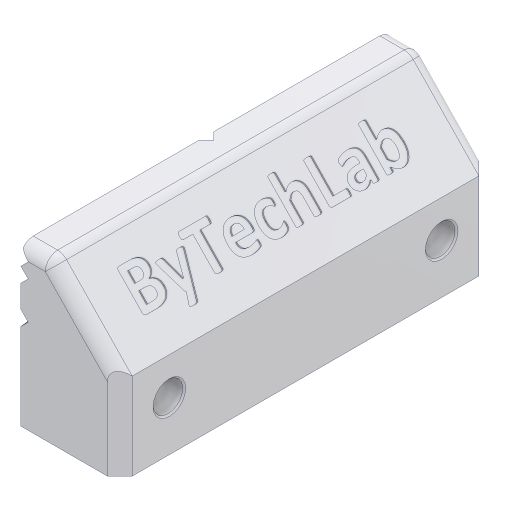
# Autodesk Inventor part: 3DP_ABS_Jaw_First_Half
Saved by Autodesk Inventor 2024.3 (Build 283343000, 343)
## iProperties
Created: 2018-02-17
Part Number: 3DP_ABS_Jaw_First_Half
Material: Ogólny
Document SubType Name: Modeling
Designer: Andrzej
Density: 1 g/cm^3
Appearance: PTFE
Author: Andrzej
Autodesk Inventor part; units mm, degrees
ref_plane "YZ Plane" through (0, 0, 0) normal (1, 0, 0) x (0, 1, 0)
ref_plane "XZ Plane" through (0, 0, 0) normal (0, 1, 0) x (-1, 0, 0)
ref_plane "XY Plane" through (0, 0, 0) normal (0, 0, 1) x (1, 0, 0)
sketch "Szkic1" plane through (0, 0, 0) normal (0, 0, 1) x (1, 0, 0)
  line L0 (-10, 37.5) -> (10, 37.5)
  line L1 (10, 37.5) -> (10, -37.5)
  line L2 (10, -37.5) -> (-10, -37.5)
  line L3 (-10, -37.5) -> (-10, 37.5)
  point P0 (0, 0)
  dimension "d0" = 20
  dimension "d1" = 75
  dimension "d39" = 37.5
  dimension "d40" = 10
  constraints: 8 end point, 2 parallel, 1 horizontal, 1 perpendicular
  measures "d0" distance of L1.end L2.end
  measures "d1" distance of L0.end L1.end
  measures "d39" distance from line of point (0, 0) L0
  measures "d40" distance from line of point (0, 0) L1
extrude "Wyciągnięcie proste1" add sketch "Szkic1" along normal blind 32
sketch "Szkic2" plane through (10, -37.5, 0) normal (1, 0, 0) x (0, 0, -1)
  line L0 (0, 75) -> (0, 0) projected
  line L1 (0, 75) -> (-32, 75) projected
  line L2 (-32, 0) -> (-32, 75) projected
  line L3 (0, 0) -> (-32, 0) projected
  point P0 (0, 37.5)
  point P1 (-10, 10)
  point P2 (-10, 65)
  dimension "d4" = 32
  dimension "d5" = 10
  dimension "d6" = 10
  dimension "d7" = 10
  dimension "d8" = 10
  measures "d4" distance of L0.end L2.start
  measures "d5" distance from line of L0 point (-10, 10)
  measures "d6" distance from line of L0 point (-10, 65)
  measures "d7" distance from line of L3 point (-10, 10)
  measures "d8" distance from line of L1 point (-10, 65)
hole "Otwór1" at (10, -27.5, 10) at (10, 27.5, 10) direction (-1, 0, 0) diameter 6 end through all
sketch "Szkic3" plane through (-10, 37.5, 0) normal (0, 1, 0) x (1, 0, 0)
  line L0 (0, 0) -> (20, 0) projected
  line L1 (0, 0) -> (0, -32) projected
  line L2 (20, -32) -> (0, -32) projected
  line L3 (20, 0) -> (20, -32) projected
  line L4 (0, -28) -> (1.5, -26.5)
  line L5 (0, -28) -> (2.2095, -28) construction
  line L6 (0, 0) -> (0, -32) projected
  line L7 (0, -25) -> (1.5, -26.5)
  line L8 (0, -25) -> (2.7592, -25) construction
  dimension "d17" = 45
  dimension "d19" = 45
  dimension "d20" = 3
  dimension "d21" = 4
  constraints: 8 end point, 2 horizontal, 2 point on line
  measures "d17" angle of L5 L4
  measures "d19" angle of L7 L8
  measures "d20" distance of L7.start L4.start
  measures "d21" distance from line of L2 L4.start
extrude "Wyciągnięcie proste2" cut sketch "Szkic3" against normal through all contours L7 L4 L1
chamfer "Faza1" distance 14 distance2 14.5 1 edges at (10, 0, 32) measured on face at (9.5, 0, 32)
chamfer "Faza2" distance 2.5 angle 45 2 edges at (10, -37.5, 8.75) (10, 37.5, 8.75)
ref_plane "Płaszczyzna konstrukcyjna1" through (-10, 37.5, 32) normal (0, -0.9902681, -0.1391731) x (-1, 0, 0)
sketch "Szkic4" plane through (-10, 37.5, 32) normal (0, -0.9902681, -0.1391731) x (-1, 0, 0)
  line L0 (-17.5, 31.6886) -> (-17.5, 11.7948) projected
  line L1 (0, 31.6886) -> (-17.5, 31.6886) projected
  line L2 (0, 31.6886) -> (0, 6.9319) projected
  line L3 (0, 6.9319) -> (-1.5, 5.4465) projected
  line L4 (-1.5, 5.4465) -> (0, 3.9611) projected
  line L5 (0, 3.9611) -> (0, 0) projected
  line L6 (-6, 0) -> (0, 0) projected
  line L7 (-17.5, 11.7948) -> (-6, 0) projected
  line L8 (0, -3.5061) -> (0, 6.9319) projected
  line L9 (0, 1) -> (-1.5, 2.5)
  line L10 (0, 1) -> (2.5951, 1) construction
  line L11 (0, 31.6886) -> (0, 6.9319) projected
  line L12 (0, 4) -> (-1.5, 2.5)
  line L13 (0, 4) -> (3.5979, 4) construction
  line L14 (0, 1) -> (0, 4)
  point P0 (-10, 26.4696)
  dimension "d32" = 135
  dimension "d34" = 135
  dimension "d35" = 3
  dimension "d36" = 1
  constraints: 10 end point, 2 horizontal, 2 point on line, 1 collinear
  measures "d32" angle of L10 L9
  measures "d34" angle of L12 L13
  measures "d35" distance of L12.start L9.start
  measures "d36" distance of L5.end L9.start
extrude "Wyciągnięcie proste3" cut sketch "Szkic4" along normal through all contours L8 L4 L12 | L9 L12 L4 L5
mirror "Odbicie lustrzane1" about plane through (0, 0, 0) normal (0, 1, 0) of "Wyciągnięcie proste3"
sketch "Szkic5" plane through (0, 0, 32) normal (0, 0, 1) x (1, 0, 0)
  line L0 (-4, 37.5) -> (-4, -37.5) projected
  line L1 (-4, 37.5) -> (-10, 37.5) projected
  line L2 (-10, 37.5) -> (-10, -37.5) projected
  line L3 (-10, -37.5) -> (-4, -37.5) projected
  line L4 (-10, 1.5) -> (-4.369, 1.5) construction
  line L5 (-10, -37.5) -> (-10, 0) projected
  line L6 (-10, -1.5) -> (-2.768, -1.5) construction
  line L7 (-10, -1.5) -> (-8.5, 0)
  line L8 (-10, 1.5) -> (-8.5, 0)
  point P0 (0, 0)
  dimension "d45" = 3
  dimension "d46" = 45
  dimension "d47" = 45
  dimension "d48" = 75
  dimension "d49" = 36
  constraints: 8 end point, 2 horizontal, 2 point on line, 1 perpendicular
  measures "d45" distance of L6.start L4.start
  measures "d46" angle of L4 L8
  measures "d47" angle of L6 L7
  measures "d48" distance of L1.end L2.end
  measures "d49" distance from line of L1 L4.start
extrude "Wyciągnięcie proste4" cut sketch "Szkic5" against normal through all contours L8 L7 L2
fillet "Zaokrąglenie1" radius 2.5 5 edges at (-4, 0, 32) (1.75, 37.5, 26.0446) (1.75, -37.5, 26.0446) (-7, -37.5, 32) (-7, 37.5, 32)
sketch "Szkic6" plane through (-10, 37.5, 0) normal (-1, 0, 0) x (0, 0, 1)
  line L0 (0, -36) -> (22.4796, -36) projected
  line L1 (22.4796, -36) -> (17.4201, 0) projected
  line L2 (0, 0) -> (17.4201, 0) projected
  line L3 (0, -36) -> (0, 0) projected
  circle A0 centre (10, -10) radius 3 projected
  line L4 (22.4796, -39) -> (0, -39) projected
  line L5 (0, -75) -> (0, -39) projected
  line L6 (0, -75) -> (17.4201, -75) projected
  line L7 (17.4201, -75) -> (22.4796, -39) projected
  circle A1 centre (10, -65) radius 3 projected
  circle A2 centre (10, -10) radius 5
  circle A3 centre (10, -65) radius 5
  line L8 (15, -12.8868) -> (10, -15.7735)
  line L9 (10, -15.7735) -> (5, -12.8868)
  line L10 (5, -12.8868) -> (5, -7.1132)
  line L11 (5, -7.1132) -> (10, -4.2265)
  line L12 (10, -4.2265) -> (15, -7.1132)
  line L13 (15, -7.1132) -> (15, -12.8868)
  line L14 (15, -67.8868) -> (10, -70.7735)
  line L15 (10, -70.7735) -> (5, -67.8868)
  line L16 (5, -67.8868) -> (5, -62.1132)
  line L17 (5, -62.1132) -> (10, -59.2265)
  line L18 (10, -59.2265) -> (15, -62.1132)
  line L19 (15, -62.1132) -> (15, -67.8868)
  point P0 (0, -37.5)
  point P1 (15, -10)
  point P2 (15, -65)
  dimension "d56" = 10
  dimension "d57" = 10
  constraints: 24 end point, 4 coincident, 2 horizontal alignment, 2 midpoint, 1 point on line, 30 other
extrude "Wyciągnięcie proste5" cut sketch "Szkic6" against normal blind 5 contours A2 | L13 L8 A2 | A2 L12 L13 | A2 L11 L12 | L8 L9 A2 | A2 L10 L11 | L9 L10 A2 | A3 | L19 L14 A3 | A3 L18 L19 | A3 L17 L18 | L14 L15 A3 | A3 L16 L17 | L15 L16 A3
chamfer "Faza4" distance 0.3 angle 45 4 edges at (-5, 27.5, 13) (10, 27.5, 13) (-5, -27.5, 13) (10, -27.5, 13)
sketch "Szkic7" plane through (-3.2628, -35, 31.2365) normal (0.7194015, 0, 0.6945945) x (0.6945945, 0, -0.7194015)
  line L0 (0, 70) -> (19.0943, 70) projected
  line L1 (0, 0) -> (0, 70) projected
  line L2 (19.0943, 0) -> (0, 0) projected
  line L3 (19.0943, 0) -> (19.0943, 70) projected
  line L4 (3.9416, 6.0812) -> (3.9416, 71.7325) construction
  line L5 (3.9416, 71.7325) -> (20.2301, 71.7325) construction
  line L6 (20.2301, 71.7325) -> (20.2301, 6.0812) construction
  line L7 (20.2301, 6.0812) -> (3.9416, 6.0812) construction
  spline S0 degree 2 poles (10.1237, 12.7216) (10.5519, 12.7216) (11.243, 12.4887) (11.7688, 12.0756) (12.1519, 11.5047) (12.3923, 10.8136) (12.5125, 10.0324) (12.5125, 9.5516) knots 0 0 0 1 2 3 4 5 6 6 6
  line L8 (12.5125, 9.5516) -> (12.5125, 7.4333)
  spline S1 degree 2 poles (12.5125, 7.4333) (12.5125, 7.2305) (12.2721, 6.9526) (12.0017, 6.9526) knots 0 0 0 1 2 2 2
  line L9 (12.0017, 6.9526) -> (5.0608, 6.9526)
  spline S2 degree 2 poles (5.0608, 6.9526) (4.7904, 6.9526) (4.55, 7.2305) (4.55, 7.4333) knots 0 0 0 1 2 2 2
  line L10 (4.55, 7.4333) -> (4.55, 9.4315)
  spline S3 degree 2 poles (4.55, 9.4315) (4.55, 10.1676) (4.7979, 11.1817) (5.2937, 11.8803) (6.0599, 12.2484) (6.5782, 12.2484) knots 0 0 0 1 2 3 4 4 4
  spline S4 degree 2 poles (6.5782, 12.2484) (6.8636, 12.2484) (7.3744, 12.0981) (7.7951, 11.8202) (8.1181, 11.407) (8.2158, 11.1366) knots 0 0 0 1 2 3 4 4 4
  spline S5 degree 2 poles (8.2158, 11.1366) (8.2759, 11.4822) (8.5838, 12.053) (9.0646, 12.4737) (9.7181, 12.7216) (10.1237, 12.7216) knots 0 0 0 1 2 3 4 4 4
  spline S6 degree 2 poles (10.1763, 11.039) (9.9059, 11.039) (9.4702, 10.8512) (9.1697, 10.4981) (9.012, 9.9422) (9.012, 9.4991) knots 0 0 0 1 2 3 4 4 4
  line L11 (9.012, 9.4991) -> (9.012, 8.5376)
  line L12 (9.012, 8.5376) -> (11.273, 8.5376)
  line L13 (11.273, 8.5376) -> (11.273, 9.7094)
  spline S7 degree 2 poles (11.273, 9.7094) (11.273, 10.0474) (11.1303, 10.5056) (10.8524, 10.8512) (10.4467, 11.039) (10.1763, 11.039) knots 0 0 0 1 2 3 4 4 4
  spline S8 degree 2 poles (6.7735, 10.6333) (6.5331, 10.6333) (6.15, 10.4831) (5.8946, 10.1901) (5.7594, 9.7394) (5.7594, 9.3563) knots 0 0 0 1 2 3 4 4 4
  line L14 (5.7594, 9.3563) -> (5.7594, 8.5376)
  line L15 (5.7594, 8.5376) -> (7.8327, 8.5376)
  line L16 (7.8327, 8.5376) -> (7.8327, 9.4465)
  spline S9 degree 2 poles (7.8327, 9.4465) (7.8327, 9.7995) (7.6674, 10.2202) (7.3744, 10.4981) (6.9838, 10.6333) (6.7735, 10.6333) knots 0 0 0 1 2 3 4 4 4
  line L17 (12.5125, 17.1009) -> (14.458, 16.4399)
  spline S10 degree 2 poles (14.458, 16.4399) (14.6082, 16.3873) (14.7435, 15.8915) (14.7435, 15.4183) knots 0 0 0 1 2 2 2
  spline S11 degree 2 poles (14.7435, 15.4183) (14.7435, 15.1704) (14.6984, 14.8775) (14.6007, 14.7272) (14.458, 14.7122) (14.3528, 14.7573) knots 0 0 0 1 2 3 4 4 4
  line L18 (14.3528, 14.7573) -> (12.5125, 15.4934)
  spline S12 degree 2 poles (12.5125, 15.4934) (12.4749, 15.4108) (12.3247, 15.2831) (12.2345, 15.253) knots 0 0 0 1 2 2 2
  line L19 (12.2345, 15.253) -> (7.1942, 13.3676)
  spline S13 degree 2 poles (7.1942, 13.3676) (6.9763, 13.285) (6.751, 13.285) (6.6233, 13.4352) (6.5707, 13.7807) (6.5707, 14.0737) knots 0 0 0 1 2 3 4 4 4
  spline S14 degree 2 poles (6.5707, 14.0737) (6.5707, 14.3366) (6.5857, 14.6446) (6.6608, 14.8174) (6.8186, 14.9075) (6.9613, 14.9526) knots 0 0 0 1 2 3 4 4 4
  line L20 (6.9613, 14.9526) -> (10.627, 16.2371)
  line L21 (10.627, 16.2371) -> (10.627, 16.2596)
  line L22 (10.627, 16.2596) -> (6.8862, 17.439)
  spline S15 degree 2 poles (6.8862, 17.439) (6.7209, 17.469) (6.6233, 17.5892) (6.5707, 17.8596) (6.5707, 18.1976) knots 0 0 0 1 2 3 3 3
  spline S16 degree 2 poles (6.5707, 18.1976) (6.5707, 18.4606) (6.6233, 18.8136) (6.7585, 18.9789) (6.9838, 18.9789) (7.1341, 18.9338) knots 0 0 0 1 2 3 4 4 4
  line L23 (7.1341, 18.9338) -> (12.5125, 17.1009)
  spline S17 degree 2 poles (5.2111, 25.2812) (5.3913, 25.2812) (5.6467, 25.2512) (5.797, 25.1911) (5.8721, 25.0934) (5.8721, 25.0408) knots 0 0 0 1 2 3 4 4 4
  line L24 (5.8721, 25.0408) -> (5.8721, 23.0502)
  line L25 (5.8721, 23.0502) -> (12.2946, 23.0502)
  spline S18 degree 2 poles (12.2946, 23.0502) (12.3547, 23.0502) (12.4524, 22.9676) (12.5125, 22.7873) (12.55, 22.4718) (12.55, 22.239) knots 0 0 0 1 2 3 4 4 4
  spline S19 degree 2 poles (12.55, 22.239) (12.55, 22.0061) (12.5125, 21.6906) (12.4524, 21.5103) (12.3547, 21.4277) (12.2946, 21.4277) knots 0 0 0 1 2 3 4 4 4
  line L26 (12.2946, 21.4277) -> (5.8721, 21.4277)
  line L27 (5.8721, 21.4277) -> (5.8721, 19.4371)
  spline S20 degree 2 poles (5.8721, 19.4371) (5.8721, 19.377) (5.797, 19.2868) (5.6467, 19.2268) (5.3913, 19.1967) (5.2111, 19.1967) knots 0 0 0 1 2 3 4 4 4
  spline S21 degree 2 poles (5.2111, 19.1967) (5.0308, 19.1967) (4.7679, 19.2268) (4.6176, 19.2868) (4.55, 19.377) (4.55, 19.4371) knots 0 0 0 1 2 3 4 4 4
  line L28 (4.55, 19.4371) -> (4.55, 25.0408)
  spline S22 degree 2 poles (4.55, 25.0408) (4.55, 25.0934) (4.6176, 25.1911) (4.7679, 25.2512) (5.0308, 25.2812) (5.2111, 25.2812) knots 0 0 0 1 2 3 4 4 4
  spline S23 degree 2 poles (9.3951, 31.2155) (9.6805, 31.2155) (9.951, 30.9601) (9.951, 30.7422) knots 0 0 0 1 2 2 2
  line L29 (9.951, 30.7422) -> (9.951, 27.3995)
  spline S24 degree 2 poles (9.951, 27.3995) (10.304, 27.3995) (10.8749, 27.5648) (11.273, 27.9329) (11.4834, 28.5038) (11.4834, 28.9019) knots 0 0 0 1 2 3 4 4 4
  spline S25 degree 2 poles (11.4834, 28.9019) (11.4834, 29.3075) (11.3632, 29.9235) (11.228, 30.3742) (11.1078, 30.6671) (11.1078, 30.7648) knots 0 0 0 1 2 3 4 4 4
  spline S26 degree 2 poles (11.1078, 30.7648) (11.1078, 30.8174) (11.1528, 30.8925) (11.258, 30.9451) (11.4608, 30.9601) (11.6186, 30.9601) knots 0 0 0 1 2 3 4 4 4
  spline S27 degree 2 poles (11.6186, 30.9601) (11.7538, 30.9601) (11.9416, 30.9451) (12.0768, 30.9225) (12.1744, 30.8775) (12.2571, 30.7948) (12.4073, 30.4343) (12.55, 29.8784) (12.6552, 29.1648) (12.6552, 28.7592) knots 0 0 0 1 2 3 4 5 6 7 8 8 8
  spline S28 degree 2 poles (12.6552, 28.7592) (12.6552, 28.0305) (12.2871, 26.9263) (11.5359, 26.1826) (10.3942, 25.8221) (9.6205, 25.8221) knots 0 0 0 1 2 3 4 4 4
  spline S29 degree 2 poles (9.6205, 25.8221) (8.8918, 25.8221) (7.7125, 26.2052) (6.8937, 26.9338) (6.4655, 27.9704) (6.4655, 28.6239) knots 0 0 0 1 2 3 4 4 4
  spline S30 degree 2 poles (6.4655, 28.6239) (6.4655, 29.315) (6.8712, 30.2915) (7.5923, 30.9225) (8.5763, 31.2155) (9.1547, 31.2155) knots 0 0 0 1 2 3 4 4 4
  line L30 (9.1547, 31.2155) -> (9.3951, 31.2155)
  spline S31 degree 2 poles (8.9519, 29.7131) (8.3059, 29.7282) (7.5622, 29.1723) (7.5622, 28.5864) knots 0 0 0 1 2 2 2
  spline S32 degree 2 poles (7.5622, 28.5864) (7.5622, 28.2934) (7.7801, 27.8577) (8.1557, 27.5648) (8.6665, 27.4145) (8.9519, 27.3995) knots 0 0 0 1 2 3 4 4 4
  line L31 (8.9519, 27.3995) -> (8.9519, 29.7131)
  spline S33 degree 2 poles (11.4308, 36.639) (11.5885, 36.639) (11.8064, 36.6239) (11.9566, 36.5864) (12.0467, 36.5488) (12.1895, 36.3986) (12.3923, 36.0455) (12.55, 35.5873) (12.6477, 35.054) (12.6477, 34.7685) knots 0 0 0 1 2 3 4 5 6 7 8 8 8
  spline S34 degree 2 poles (12.6477, 34.7685) (12.6477, 34.1376) (12.2571, 33.1535) (11.4834, 32.4925) (10.3791, 32.1545) (9.658, 32.1545) knots 0 0 0 1 2 3 4 4 4
  spline S35 degree 2 poles (9.658, 32.1545) (8.8392, 32.1545) (7.6374, 32.5676) (6.8486, 33.3038) (6.4655, 34.3103) (6.4655, 34.9188) knots 0 0 0 1 2 3 4 4 4
  spline S36 degree 2 poles (6.4655, 34.9188) (6.4655, 35.1592) (6.5557, 35.6399) (6.6984, 36.0455) (6.8862, 36.3761) (7.0214, 36.5113) (7.1115, 36.5638) (7.2618, 36.5939) (7.4796, 36.6164) (7.6298, 36.6164) knots 0 0 0 1 2 3 4 5 6 7 8 8 8
  spline S37 degree 2 poles (7.6298, 36.6164) (7.9904, 36.6164) (8.2759, 36.4887) (8.2759, 36.3911) knots 0 0 0 1 2 2 2
  spline S38 degree 2 poles (8.2759, 36.3911) (8.2759, 36.2859) (8.1031, 36.053) (7.8928, 35.7376) (7.72, 35.2944) (7.72, 34.9864) knots 0 0 0 1 2 3 4 4 4
  spline S39 degree 2 poles (7.72, 34.9864) (7.72, 34.3779) (8.6514, 33.7394) (9.5528, 33.7394) knots 0 0 0 1 2 2 2
  spline S40 degree 2 poles (9.5528, 33.7394) (9.996, 33.7394) (10.6721, 33.8972) (11.1303, 34.2127) (11.3557, 34.6859) (11.3557, 35.0014) knots 0 0 0 1 2 3 4 4 4
  spline S41 degree 2 poles (11.3557, 35.0014) (11.3557, 35.3244) (11.1679, 35.7826) (10.9275, 36.1282) (10.7397, 36.361) (10.7397, 36.4437) knots 0 0 0 1 2 3 4 4 4
  spline S42 degree 2 poles (10.7397, 36.4437) (10.7397, 36.4962) (10.7998, 36.5714) (10.9651, 36.6164) (11.228, 36.639) (11.4308, 36.639) knots 0 0 0 1 2 3 4 4 4
  spline S43 degree 2 poles (12.3021, 43.0014) (12.3622, 43.0014) (12.4599, 42.9263) (12.52, 42.7535) (12.55, 42.453) (12.55, 42.2277) knots 0 0 0 1 2 3 4 4 4
  spline S44 degree 2 poles (12.55, 42.2277) (12.55, 42.0023) (12.52, 41.7019) (12.4599, 41.5291) (12.3622, 41.454) (12.3021, 41.454) knots 0 0 0 1 2 3 4 4 4
  line L32 (12.3021, 41.454) -> (9.1697, 41.454)
  spline S45 degree 2 poles (9.1697, 41.454) (8.7716, 41.454) (8.3134, 41.3338) (7.9904, 41.116) (7.8101, 40.7629) (7.8101, 40.53) knots 0 0 0 1 2 3 4 4 4
  spline S46 degree 2 poles (7.8101, 40.53) (7.8101, 40.2371) (8.2383, 39.6286) (8.6514, 39.3056) knots 0 0 0 1 2 2 2
  line L33 (8.6514, 39.3056) -> (12.3021, 39.3056)
  spline S47 degree 2 poles (12.3021, 39.3056) (12.3622, 39.3056) (12.4599, 39.2305) (12.52, 39.0502) (12.55, 38.7573) (12.55, 38.5319) knots 0 0 0 1 2 3 4 4 4
  spline S48 degree 2 poles (12.55, 38.5319) (12.55, 38.3066) (12.52, 38.0136) (12.4599, 37.8333) (12.3622, 37.7582) (12.3021, 37.7582) knots 0 0 0 1 2 3 4 4 4
  line L34 (12.3021, 37.7582) -> (4.2045, 37.7582)
  spline S49 degree 2 poles (4.2045, 37.7582) (4.1444, 37.7582) (4.0467, 37.8333) (3.9791, 38.0136) (3.9416, 38.3066) (3.9416, 38.5319) knots 0 0 0 1 2 3 4 4 4
  spline S50 degree 2 poles (3.9416, 38.5319) (3.9416, 38.7573) (3.9791, 39.0502) (4.0467, 39.2305) (4.1444, 39.3056) (4.2045, 39.3056) knots 0 0 0 1 2 3 4 4 4
  line L35 (4.2045, 39.3056) -> (7.2467, 39.3056)
  spline S51 degree 2 poles (7.2467, 39.3056) (6.8561, 39.7038) (6.4655, 40.5376) (6.4655, 40.9883) knots 0 0 0 1 2 2 2
  spline S52 degree 2 poles (6.4655, 40.9883) (6.4655, 41.5441) (6.8336, 42.3178) (7.4721, 42.7911) (8.3284, 43.0014) (8.9369, 43.0014) knots 0 0 0 1 2 3 4 4 4
  line L36 (8.9369, 43.0014) -> (12.3021, 43.0014)
  spline S53 degree 2 poles (11.8364, 48.9958) (12.0167, 48.9958) (12.2721, 48.9657) (12.4374, 48.9056) (12.5125, 48.808) (12.5125, 48.7479) knots 0 0 0 1 2 3 4 4 4
  line L37 (12.5125, 48.7479) -> (12.5125, 45.0972)
  spline S54 degree 2 poles (12.5125, 45.0972) (12.5125, 44.8944) (12.2721, 44.6164) (12.0017, 44.6164) knots 0 0 0 1 2 2 2
  line L38 (12.0017, 44.6164) -> (4.7679, 44.6164)
  spline S55 degree 2 poles (4.7679, 44.6164) (4.7078, 44.6164) (4.6101, 44.6991) (4.55, 44.8793) (4.5125, 45.1948) (4.5125, 45.4277) knots 0 0 0 1 2 3 4 4 4
  spline S56 degree 2 poles (4.5125, 45.4277) (4.5125, 45.6681) (4.55, 45.9761) (4.6101, 46.1563) (4.7078, 46.239) (4.7679, 46.239) knots 0 0 0 1 2 3 4 4 4
  line L39 (4.7679, 46.239) -> (11.1754, 46.239)
  line L40 (11.1754, 46.239) -> (11.1754, 48.7479)
  spline S57 degree 2 poles (11.1754, 48.7479) (11.1754, 48.808) (11.243, 48.9056) (11.4007, 48.9657) (11.6486, 48.9958) (11.8364, 48.9958) knots 0 0 0 1 2 3 4 4 4
  spline S58 degree 2 poles (12.3247, 54.5319) (12.4073, 54.5319) (12.505, 54.4117) (12.55, 54.1413) (12.55, 53.8859) knots 0 0 0 1 2 3 3 3
  spline S59 degree 2 poles (12.55, 53.8859) (12.55, 53.608) (12.505, 53.3601) (12.4073, 53.2549) (12.3247, 53.2549) knots 0 0 0 1 2 3 3 3
  line L41 (12.3247, 53.2549) -> (11.8815, 53.2549)
  spline S60 degree 2 poles (11.8815, 53.2549) (12.2496, 52.9169) (12.6552, 52.0455) (12.6552, 51.5197) knots 0 0 0 1 2 2 2
  spline S61 degree 2 poles (12.6552, 51.5197) (12.6552, 51.0765) (12.4298, 50.3479) (11.9791, 49.807) (11.3181, 49.5141) (10.8749, 49.5141) knots 0 0 0 1 2 3 4 4 4
  spline S62 degree 2 poles (10.8749, 49.5141) (10.3942, 49.5141) (9.6881, 49.8897) (9.2223, 50.6333) (9.0045, 51.7451) (9.0045, 52.4812) knots 0 0 0 1 2 3 4 4 4
  line L42 (9.0045, 52.4812) -> (9.0045, 53.0145)
  line L43 (9.0045, 53.0145) -> (8.674, 53.0145)
  spline S63 degree 2 poles (8.674, 53.0145) (8.4111, 53.0145) (8.0205, 52.9094) (7.7575, 52.669) (7.6374, 52.2709) (7.6374, 51.9704) knots 0 0 0 1 2 3 4 4 4
  spline S64 degree 2 poles (7.6374, 51.9704) (7.6374, 51.5873) (7.8101, 50.9714) (8.0205, 50.5056) (8.1932, 50.1901) (8.1932, 50.0925) knots 0 0 0 1 2 3 4 4 4
  spline S65 degree 2 poles (8.1932, 50.0925) (8.1932, 50.0249) (8.1106, 49.9197) (7.9453, 49.8521) (7.7125, 49.8145) (7.5697, 49.8145) knots 0 0 0 1 2 3 4 4 4
  spline S66 degree 2 poles (7.5697, 49.8145) (7.382, 49.8145) (7.1641, 49.8746) (6.9838, 50.0474) (6.766, 50.4831) (6.5857, 51.0615) (6.4655, 51.7451) (6.4655, 52.1056) knots 0 0 0 1 2 3 4 5 6 6 6
  spline S67 degree 2 poles (6.4655, 52.1056) (6.4655, 52.7516) (6.7209, 53.6681) (7.2392, 54.2615) (8.0655, 54.5319) (8.6289, 54.5319) knots 0 0 0 1 2 3 4 4 4
  line L44 (8.6289, 54.5319) -> (12.3247, 54.5319)
  line L45 (9.9735, 53.0145) -> (9.9735, 52.4211)
  spline S68 degree 2 poles (9.9735, 52.4211) (9.9735, 52.0455) (10.0862, 51.5197) (10.304, 51.1892) (10.6195, 51.0315) (10.8223, 51.0315) knots 0 0 0 1 2 3 4 4 4
  spline S69 degree 2 poles (10.8223, 51.0315) (11.1679, 51.0315) (11.5585, 51.4671) (11.5585, 51.8577) knots 0 0 0 1 2 2 2
  spline S70 degree 2 poles (11.5585, 51.8577) (11.5585, 52.1807) (11.228, 52.7291) (10.905, 53.0145) knots 0 0 0 1 2 2 2
  line L46 (10.905, 53.0145) -> (9.9735, 53.0145)
  spline S71 degree 2 poles (9.4852, 61.6005) (10.2214, 61.6005) (11.3857, 61.2775) (12.212, 60.6765) (12.6552, 59.7976) (12.6552, 59.2343) knots 0 0 0 1 2 3 4 4 4
  spline S72 degree 2 poles (12.6552, 59.2343) (12.6552, 58.9563) (12.55, 58.4756) (12.3172, 58.0399) (11.9566, 57.6117) (11.7087, 57.3939) knots 0 0 0 1 2 3 4 4 4
  line L47 (11.7087, 57.3939) -> (12.3021, 57.3939)
  spline S73 degree 2 poles (12.3021, 57.3939) (12.3697, 57.3939) (12.4674, 57.3263) (12.5275, 57.1685) (12.55, 56.9131) (12.55, 56.7253) knots 0 0 0 1 2 3 4 4 4
  spline S74 degree 2 poles (12.55, 56.7253) (12.55, 56.5376) (12.5275, 56.2897) (12.4674, 56.1319) (12.3697, 56.0718) (12.3021, 56.0718) knots 0 0 0 1 2 3 4 4 4
  line L48 (12.3021, 56.0718) -> (4.2045, 56.0718)
  spline S75 degree 2 poles (4.2045, 56.0718) (4.1444, 56.0718) (4.0467, 56.1469) (3.9791, 56.3272) (3.9416, 56.6202) (3.9416, 56.8455) knots 0 0 0 1 2 3 4 4 4
  spline S76 degree 2 poles (3.9416, 56.8455) (3.9416, 57.0709) (3.9791, 57.3638) (4.0467, 57.5441) (4.1444, 57.6192) (4.2045, 57.6192) knots 0 0 0 1 2 3 4 4 4
  line L49 (4.2045, 57.6192) -> (7.2467, 57.6192)
  spline S77 degree 2 poles (7.2467, 57.6192) (7.0364, 57.8296) (6.7435, 58.2502) (6.5482, 58.6634) (6.4655, 59.1141) (6.4655, 59.3545) knots 0 0 0 1 2 3 4 4 4
  spline S78 degree 2 poles (6.4655, 59.3545) (6.4655, 59.9704) (6.9538, 60.8192) (7.7726, 61.3526) (8.8768, 61.6005) (9.4852, 61.6005) knots 0 0 0 1 2 3 4 4 4
  spline S79 degree 2 poles (9.5979, 59.993) (9.2449, 59.993) (8.5913, 59.8878) (8.0881, 59.6324) (7.7876, 59.2192) (7.7876, 58.9038) knots 0 0 0 1 2 3 4 4 4
  spline S80 degree 2 poles (7.7876, 58.9038) (7.7876, 58.746) (7.8702, 58.453) (8.0805, 58.1376) (8.4186, 57.807) (8.6589, 57.6192) knots 0 0 0 1 2 3 4 4 4
  line L50 (8.6589, 57.6192) -> (10.4843, 57.6192)
  spline S81 degree 2 poles (10.4843, 57.6192) (10.905, 57.9498) (11.3406, 58.5432) (11.3406, 58.8737) knots 0 0 0 1 2 2 2
  spline S82 degree 2 poles (11.3406, 58.8737) (11.3406, 59.1742) (11.0327, 59.5948) (10.5369, 59.8728) (9.9134, 59.993) (9.5979, 59.993) knots 0 0 0 1 2 3 4 4 4
  point P0 (24.7379, 35)
  constraints: 2 other
extrude "Wyciągnięcie proste6" cut sketch "Szkic7" against normal blind 0.3 contours S0 L8 S1 L9 S2 L10 S3 S4 S5 | L17 S10 S11 L18 S12 L19 S13 S14 L20 L21 L22 S15 S16 L23 | S17 L24 L25 S18 S19 L26 L27 S20 S21 L28 S22 | S23 L29 S24 S25 S26 S27 S28 S29 S30 L30 | S33 S34 S35 S36 S37 S38 S39 S40 S41 S42 | S43 S44 L32 S45 S46 L33 S47 S48 L34 S49 S50 L35 S51 S52 L36 | S53 L37 S54 L38 S55 S56 L39 L40 S57 | S58 S59 L41 S60 S61 S62 L42 L43 S63 S64 S65 S66 S67 L44 | S71 S72 L47 S73 S74 L48 S75 S76 L49 S77 S78
sketch "Szkic8" plane through (0, 0, 0) normal (0, 0, -1) x (-1, 0, 0)
  circle A0 centre (0, 0) radius 5
  line L0 (10, -1.5) -> (8.5, 0) projected
  line L1 (8.5, 0) -> (10, 1.5) projected
  line L2 (10, 1.5) -> (10, 37.5) projected
  line L3 (10, 37.5) -> (-7.5, 37.5) projected
  line L4 (-10, 35) -> (-7.5, 37.5) projected
  line L5 (-10, 35) -> (-10, -35) projected
  line L6 (-7.5, -37.5) -> (-10, -35) projected
  line L7 (-7.5, -37.5) -> (10, -37.5) projected
  line L8 (10, -37.5) -> (10, -1.5) projected
  point P0 (0, 0)
  dimension "d65" = 10
  dimension "d66" = 75
  dimension "d67" = 20
  dimension "d68" = 10
  dimension "d69" = 37.5
  constraints: 1 centre point
  measures "d65" diameter of A0
  measures "d66" distance between parallel lines of L3 L7
  measures "d67" distance between parallel lines of L5 L2
  measures "d68" distance from line of L2 A0.centre
  measures "d69" distance from line of L7 point (0, 0)
extrude "Wyciągnięcie proste7" cut sketch "Szkic8" against normal blind 4.2 contours A0
chamfer "Faza5" distance 0.3 angle 45 1 edges at (5, 0, 0)
equation "\"d39\" = 0.5 * d1"
equation "\"d40\" = 0.5 * d0"
equation "\"d6\" = d5"
equation "\"d8\" = d7"
equation "\"d49\" = -0.5 * d45 + 0.5 * d48"
equation "\"d68\" = 0.5 * d67"
